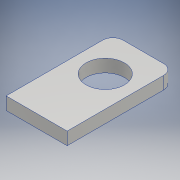
# Autodesk Inventor part: 베어링받침대
Saved by Autodesk Inventor 2017 (Build 210142000, 142)
## iProperties
Part Number: 베어링받침대
Material: 알루미늄 6061
Document SubType Name: Modeling
Designer: minom
Density: 2.7 g/cm^3
Appearance: 알루미늄 - 평지
Mass: 11.0977 g
Surface Area: 25.2413 cm^2
Volume: 4.11027 cm^3
Author: minom
Autodesk Inventor part; units mm, degrees
ref_plane "YZ Plane" through (0, 0, 0) normal (1, 0, 0) x (0, 1, 0)
ref_plane "XZ Plane" through (0, 0, 0) normal (0, 1, 0) x (-1, 0, 0)
ref_plane "XY Plane" through (0, 0, 0) normal (0, 0, 1) x (1, 0, 0)
sketch "스케치1" plane through (0, 0, 0) normal (0, 0, 1) x (1, 0, 0)
  line L0 (0, 0) -> (-24, 0)
  line L1 (-24, 0) -> (-24, 38)
  line L2 (-20, 42) -> (-4, 42)
  line L3 (0, 38) -> (0, 0)
  arc A0 (0, 38) -> (-4, 42) centre (-4, 38) ccw
  arc A1 (-20, 42) -> (-24, 38) centre (-20, 38) ccw
  circle A2 centre (-12, 27) radius 7.55
  point P0 (-24, 42)
  point P1 (0, 42)
  dimension "d0" = 24
  dimension "d1" = 42
  dimension "d2" = 4
  dimension "d4" = 15.1
  constraints: 8 end point, 4 point on circle, 4 point on line, 4 tangent, 3 centre point, 2 parallel, 1 equal radius, 1 horizontal, 1 perpendicular
  measures "d0" distance of point (-24, 42) point (0, 42)
  measures "d1" distance of L0.end point (-24, 42)
  measures "d2" radius of A0
  measures "d4" diameter of A2
extrude "돌출1" add sketch "스케치1" along normal blind 5
